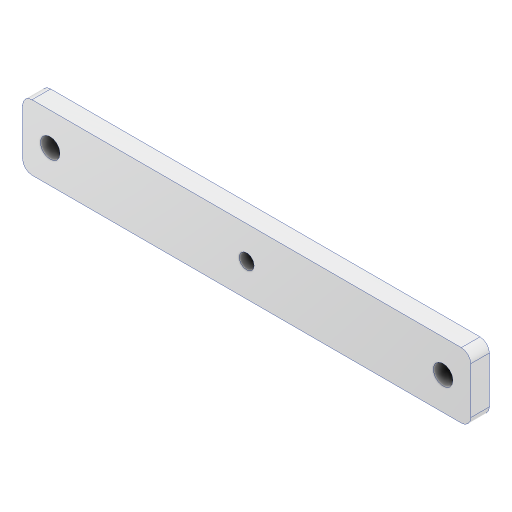
# Autodesk Inventor part: 축지지프레임
Saved by Autodesk Inventor 2023.2 (Build 272271000, 271)
## iProperties
Created: 2022-12-28
Part Number: 축지지프레임
Material: 알루미늄 6061
Document SubType Name: Modeling
Designer: BAEK
Density: 2.7 g/cm^3
Appearance: 알루미늄 - 평지
Mass: 26.5576 g
Surface Area: 61.713 cm^2
Volume: 9.83616 cm^3
Author: BAEK
Autodesk Inventor part; units mm, degrees
ref_plane "YZ Plane" through (0, 0, 0) normal (1, 0, 0) x (0, 1, 0)
ref_plane "XZ Plane" through (0, 0, 0) normal (0, 1, 0) x (-1, 0, 0)
ref_plane "XY Plane" through (0, 0, 0) normal (0, 0, 1) x (1, 0, 0)
sketch "스케치1" plane through (0, 0, 0) normal (0, 0, 1) x (1, 0, 0)
  line L0 (-48, 7) -> (48, 7)
  line L1 (48, 7) -> (48, -7)
  line L2 (48, -7) -> (-48, -7)
  line L3 (-48, -7) -> (-48, 7)
  line L4 (-48, 7) -> (48, -7) construction
  line L5 (48, 7) -> (-48, -7) construction
  point P0 (0, 0)
  dimension "d0" = 96
  dimension "d1" = 14
  constraints: 12 end point, 2 midpoint, 2 parallel, 1 horizontal, 1 perpendicular
  measures "d0" distance of L1.end L2.end
  measures "d1" distance of L0.end L1.end
extrude "돌출1" add sketch "스케치1" along normal blind 4
sketch "스케치2" plane through (0, 0, 4) normal (0, 0, 1) x (1, 0, 0)
  line L0 (-48, -7) -> (48, -7) projected
  line L1 (48, -7) -> (48, 7) projected
  line L2 (48, 7) -> (-48, 7) projected
  line L3 (-48, 7) -> (-48, -7) projected
  circle A0 centre (-42.1, 0) radius 2.1
  circle A1 centre (42.1, 0) radius 2.1
  point P0 (0, 0)
  dimension "d4" = 4.2
  dimension "d5" = 4.2
  dimension "d6" = 84.2
  dimension "d7" = 5.9
  dimension "d10" = 7
  constraints: 2 centre point, 1 horizontal alignment
  measures "d4" diameter of A0
  measures "d5" diameter of A1
  measures "d6" distance of A0.centre A1.centre
  measures "d7" distance from line of L3 A0.centre
  measures "d10" distance from line of L0 A0.centre
extrude "돌출2" cut sketch "스케치2" against normal blind 4 contours A0 | A1
fillet "모깎기1" radius 2 4 edges at (48, 7, 2) (48, -7, 2) (-48, 7, 2) (-48, -7, 2)
sketch "스케치3" plane through (0, 0, 4) normal (0, 0, 1) x (1, 0, 0)
  circle A0 centre (0, 0) radius 1.6
  dimension "d12" = 3.2
  constraints: 1 centre point, 1 coincident
  measures "d12" diameter of A0
extrude "돌출3" cut sketch "스케치3" against normal blind 4
sketch "스케치5" plane through (0, 0, 4) normal (0, 0, 1) x (1, 0, 0)
  circle A0 centre (0, 0) radius 1.6 projected
  arc A1 (-48, -5) -> (-46, -7) centre (-46, -5) ccw projected
  line L0 (-46, -7) -> (46, -7) projected
  arc A2 (46, -7) -> (48, -5) centre (46, -5) ccw projected
  line L1 (48, -5) -> (48, 5) projected
  arc A3 (48, 5) -> (46, 7) centre (46, 5) ccw projected
  line L2 (46, 7) -> (-46, 7) projected
  arc A4 (-46, 7) -> (-48, 5) centre (-46, 5) ccw projected
  line L3 (-48, 5) -> (-48, -5) projected
  circle A5 centre (42.1, 0) radius 2.1 projected
  circle A6 centre (-42.1, 0) radius 2.1 projected
  arc A7 (-46, 7) -> (-48, 5) centre (-46, 5) ccw projected
  line L4 (-48, 5) -> (-48, 20)
  line L5 (-44, 24) -> (44, 24)
  arc A8 (48, 5) -> (46, 7) centre (46, 5) ccw projected
  line L6 (48, 20) -> (48, 5)
  arc A9 (-44, 24) -> (-48, 20) centre (-44, 20) ccw
  arc A10 (48, 20) -> (44, 24) centre (44, 20) ccw
  point P0 (-48, 24)
  point P1 (48, 24)
  dimension "d18" = 19
  dimension "d21" = 4
  constraints: 6 end point, 6 tangent, 4 point on circle, 4 point on line, 2 centre point, 2 perpendicular, 1 equal radius, 1 vertical
  measures "d18" distance of L3.start point (-48, 24)
  measures "d21" radius of A9
sketch "스케치6" plane through (0, 0, 4) normal (0, 0, 1) x (1, 0, 0)
  circle A0 centre (0, 0) radius 1.6 projected
  arc A1 (-48, -5) -> (-46, -7) centre (-46, -5) ccw projected
  line L0 (-46, -7) -> (46, -7) projected
  arc A2 (46, -7) -> (48, -5) centre (46, -5) ccw projected
  line L1 (48, -5) -> (48, 20) projected
  arc A3 (48, 20) -> (44, 24) centre (44, 20) ccw projected
  line L2 (44, 24) -> (-44, 24) projected
  arc A4 (-44, 24) -> (-48, 20) centre (-44, 20) ccw projected
  line L3 (-48, 20) -> (-48, -5) projected
  circle A5 centre (42.1, 0) radius 2.1 projected
  circle A6 centre (-42.1, 0) radius 2.1 projected
  line L4 (48, -5) -> (48, 20) projected
  line L5 (-48, 23.602) -> (48, 23.602)
  line L6 (48, 23.602) -> (48, 18)
  line L7 (48, 18) -> (-48, 18)
  line L8 (-48, 18) -> (-48, 23.602)
  circle A7 centre (0, 20.4) radius 1.6
  circle A8 centre (-42.1, 20.4) radius 1.6
  circle A9 centre (42.1, 20.4) radius 1.6
  dimension "d23" = 3.2
  dimension "d24" = 3.2
  dimension "d35" = 3.6
  constraints: 8 end point, 3 centre point, 2 horizontal alignment, 2 parallel, 1 horizontal, 1 perpendicular, 1 point on line
  measures "d23" diameter of A8
  measures "d24" diameter of A9
  measures "d35" distance from line of L2 A9.centre
sketch "스케치8" plane through (0, 0, 0) normal (0, 0, -1) x (-1, 0, 0)
  circle A0 centre (-42.1, 20.4) radius 1.6 projected
  circle A1 centre (0, 20.4) radius 1.6 projected
  circle A2 centre (42.1, 20.4) radius 1.6 projected
  circle A3 centre (0, 0) radius 1.6 projected
  circle A4 centre (-42.1, 0) radius 2.1 projected
  circle A5 centre (42.1, 0) radius 2.1 projected
  arc A6 (46, -7) -> (48, -5) centre (46, -5) ccw projected
  line L0 (48, 20) -> (48, -5) projected
  arc A7 (48, 20) -> (44, 24) centre (44, 20) ccw projected
  line L1 (44, 24) -> (-44, 24) projected
  arc A8 (-44, 24) -> (-48, 20) centre (-44, 20) ccw projected
  line L2 (-48, 20) -> (-48, -5) projected
  arc A9 (-48, -5) -> (-46, -7) centre (-46, -5) ccw projected
  line L3 (46, -7) -> (-46, -7) projected
  line L4 (-48, 24) -> (-18, 24)
  line L5 (-18, 24) -> (-18, 9)
  line L6 (-18, 9) -> (-48, 9)
  line L7 (-48, 9) -> (-48, 24)
  point P0 (-44, 24)
  dimension "d27" = 30
  dimension "d28" = 15
  constraints: 8 end point, 2 parallel, 1 horizontal, 1 perpendicular
  measures "d27" distance of L5.end L6.end
  measures "d28" distance of L4.end L5.end
sketch "스케치10" plane through (0, 0, 0) normal (0, 0, -1) x (-1, 0, 0)
  arc A0 (-45, 9) -> (-48, 6) centre (-45, 6) ccw projected
  line L0 (-48, 6) -> (-48, -5) projected
  arc A1 (-48, -5) -> (-46, -7) centre (-46, -5) ccw projected
  line L1 (46, -7) -> (-46, -7) projected
  arc A2 (46, -7) -> (48, -5) centre (46, -5) ccw projected
  line L2 (48, 20) -> (48, -5) projected
  arc A3 (48, 20) -> (44, 24) centre (44, 20) ccw projected
  line L3 (44, 24) -> (-15, 24) projected
  arc A4 (-15, 24) -> (-18, 21) centre (-15, 21) ccw projected
  line L4 (-18, 21) -> (-18, 12) projected
  arc A5 (-21, 9) -> (-18, 12) centre (-21, 12) ccw projected
  line L5 (-21, 9) -> (-45, 9) projected
  circle A6 centre (42.1, 0) radius 2.1 projected
  circle A7 centre (-42.1, 0) radius 2.1 projected
  circle A8 centre (0, 0) radius 1.6 projected
  circle A9 centre (42.1, 20.4) radius 1.6 projected
  circle A10 centre (0, 20.4) radius 1.6 projected
  circle A11 centre (21.05, 20.4) radius 1.6
  dimension "d32" = 21.05
  constraints: 1 centre point, 1 equal radius
  measures "d32" distance of A10.centre A11.centre
